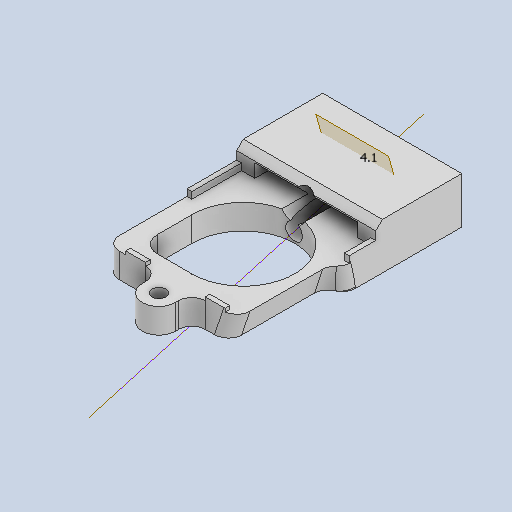
# Autodesk Inventor part: chamber bottom seal plate
Saved by Autodesk Inventor 2023.3 (Build 273359000, 359)
## iProperties
Created: 2023-03-28
Part Number: chamber bottom seal plate
Material: Generic
Document SubType Name: Modeling
Designer: splath
Density: 1 g/cm^3
Appearance: Default
Author: splath
Autodesk Inventor part; units mm, degrees
ref_plane "YZ Plane" through (0, 0, 0) normal (1, 0, 0) x (0, 1, 0)
ref_plane "XZ Plane" through (0, 0, 0) normal (0, 1, 0) x (-1, 0, 0)
ref_plane "XY Plane" through (0, 0, 0) normal (0, 0, 1) x (1, 0, 0)
sketch "Sketch1" plane through (0, 0, 0) normal (0, 0, 1) x (1, 0, 0)
  line L0 (-29.4, 0) -> (29.4, 0) construction
  line L1 (0, -2.8) -> (0, 16.8) construction
  line L2 (-21, 14) -> (21, 14)
  line L3 (21, 14) -> (21, 0)
  line L4 (21, 0) -> (-21, 0)
  line L5 (-21, 0) -> (-21, 14)
  point P0 (0, 0)
  dimension "d0" = 42
  dimension "d1" = 14
  constraints: 8 end point, 2 parallel, 1 horizontal, 1 midpoint, 1 perpendicular
  measures "d0" distance of L2.start L2.end
  measures "d1" distance of L2.end L3.end
extrude "Extrusion1" add sketch "Sketch1" along normal blind 65.5
sketch "Sketch2" plane through (0, 0, 0) normal (0, 0, -1) x (-1, 0, 0)
  line L0 (-11.5, 5) -> (11.5, 5) construction
  line L1 (0, -2.8) -> (0, 16.8) construction
  line L2 (-21, 14) -> (21, 14) construction
  line L3 (0, 5) -> (0, 0) construction
  dimension "d5" = 9
  dimension "d6" = 23
  constraints: 4 end point, 2 coincident, 1 horizontal, 1 midpoint, 1 vertical
  measures "d5" distance between parallel lines of L2 L0
  measures "d6" distance of L0.start L0.end
hole "Hole1" at (-11.5, 5, 0) at (11.5, 5, 0) direction (0, 0, 1) diameter 2.95 depth 8 tip angle 118
sketch "Sketch4" plane through (-21, 14, 0) normal (0, 1, 0) x (1, 0, 0)
  line L0 (42, 0) -> (0, 0) construction
  line L1 (0, 0) -> (0, -65.5) construction
  line L2 (42, -65.5) -> (0, -65.5) construction
  line L3 (42, 0) -> (42, -65.5) construction
  line L4 (0, -26) -> (42, -26)
  line L5 (42, -26) -> (42, -65.5)
  line L6 (42, -65.5) -> (0, -65.5)
  line L7 (0, -65.5) -> (0, -26)
  point P0 (21, 0)
  dimension "d22" = 26
  constraints: 8 end point, 3 collinear, 2 parallel, 1 horizontal, 1 perpendicular
  measures "d22" distance between parallel lines of L0 L4
extrude "Extrusion2" cut sketch "Sketch4" against normal blind 4.5
sketch "Sketch5" plane through (-21, 0, 0) normal (0, -1, 0) x (1, 0, 0)
  line L0 (0, 0) -> (42, 0) construction
  line L1 (42, 0) -> (42, 65.5) construction
  line L2 (0, 65.5) -> (42, 65.5) construction
  line L3 (0, 0) -> (0, 65.5) construction
  line L4 (21, 0) -> (21, 45) construction
  dimension "d25" = 45
  constraints: 2 end point, 1 vertical
  measures "d25" distance of L4.start L4.end
hole "Hole3" at (0, 0, 45) direction (0, 1, 0) diameter 31 end through all
sketch "Sketch6" plane through (-21, 9.5, 0) normal (0, 1, 0) x (1, 0, 0)
  line L0 (1.45, -64.1) -> (40.55, -64.1)
  line L1 (40.55, -64.1) -> (40.55, -26)
  line L2 (40.55, -26) -> (1.45, -26)
  line L3 (1.45, -26) -> (1.45, -64.1)
  line L4 (0, -26) -> (42, -26) construction
  line L5 (42, -26) -> (42, -65.5) construction
  line L6 (0, -65.5) -> (0, -26) construction
  line L7 (1.45, -41) -> (0, -41)
  line L8 (0, -41) -> (0, -65.5)
  line L9 (0, -65.5) -> (6, -65.5)
  line L10 (6, -65.5) -> (6, -64.1)
  line L11 (36, -64.1) -> (36, -65.5)
  line L12 (36, -65.5) -> (42, -65.5)
  line L13 (42, -65.5) -> (42, -34)
  line L14 (40.55, -34) -> (42, -34)
  line L15 (12, -65.5) -> (30, -65.5)
  line L16 (30, -65.5) -> (30, -64.1)
  line L17 (30, -64.1) -> (12, -64.1)
  line L18 (12, -64.1) -> (12, -65.5)
  line L19 (42, -65.5) -> (0, -65.5) construction
  point P0 (21, 0)
  point P1 (39, -65.5)
  point P2 (21, -64.1)
  dimension "d33" = 1.45
  dimension "d34" = 1.45
  dimension "d37" = 1.4
  dimension "d38" = 8
  dimension "d50" = 6
  dimension "d66" = 18
  dimension "d93" = 15
  constraints: 32 end point, 7 point on line, 5 parallel, 5 perpendicular, 4 collinear, 3 horizontal, 3 midpoint
  measures "d33" distance between parallel lines of L1 L5
  measures "d34" distance between parallel lines of L6 L3
  measures "d37" distance from line of point (39, -65.5) L0
  measures "d38" distance between parallel lines of L4 L14
  measures "d50" distance between parallel lines of L13 L11
  measures "d66" distance between parallel lines of L16 L18
  measures "d93" distance between parallel lines of L4 L7
extrude "Extrusion3" cut sketch "Sketch6" against normal blind 2
sketch "Sketch3" plane through (-0.5, -1, 34) normal (0, 0, 1) x (1, 0, 0)
  line L0 (-20.5, 1) -> (21.5, 1) construction
  line L1 (21.5, 1) -> (21.5, 8.5) construction
  line L2 (-20.5, 8.5) -> (-20.5, 1) construction
  line L3 (-8.5, 10.5) -> (-14.5, 10.5) projected
  line L4 (-14.5, 8.5) -> (-20.5, 8.5) projected
  line L5 (21.5, 8.5) -> (15.5, 8.5) projected
  line L6 (15.5, 8.5) -> (15.5, 10.5) projected
  line L7 (-14.5, 10.5) -> (-14.5, 8.5) projected
  line L8 (15.5, 10.5) -> (9.5, 10.5) projected
  line L9 (9.5, 10.5) -> (9.5, 8.5) projected
  line L10 (9.5, 8.5) -> (-8.5, 8.5) projected
  line L11 (-8.5, 8.5) -> (-8.5, 10.5) projected
  line L12 (0.5, 10) -> (0.5, 1) construction
  line L13 (21.5, 15) -> (-20.5, 15) construction
  dimension "d76" = 5
  constraints: 2 end point, 1 vertical
  measures "d76" distance from line of L12.start L13
hole "Hole2" at (0, 9, 34) direction (0, 0, -1) diameter 4.6 end through all counterbore diameter 7.5 counterbore depth 29
sketch "Sketch7" plane through (-21, 7.5, 0) normal (0, 1, 0) x (1, 0, 0)
  arc A0 (17.5631, -29.8859) -> (24.4369, -29.8859) centre (21, -45) ccw construction
  line L0 (2.9, -45) -> (39.1, -45) construction
  line L1 (0, -65.5) -> (0, -41) construction
  point P0 (21, 0)
  point P1 (21, -45)
  dimension "d49" = 2.9
  constraints: 2 coincident, 2 end point, 1 horizontal, 1 midpoint
  measures "d49" distance from line of L1 L0.start
feature "Snap Fit1" [suppressed]
fillet "Fillet1" [suppressed]
sketch "Sketch8" plane through (-21, 9.5, 0) normal (0, 1, 0) x (1, 0, 0)
  line L0 (-3.5583, -70.8259) -> (42.547, -70.8259)
  line L1 (42.547, -70.8259) -> (42.547, -58.9679)
  line L2 (42.547, -58.9679) -> (-3.5583, -58.9679)
  line L3 (-3.5583, -58.9679) -> (-3.5583, -70.8259)
  point P0 (21, 0)
  constraints: 8 end point, 2 parallel, 1 horizontal, 1 perpendicular
extrude "Extrusion4" cut sketch "Sketch8" against normal blind 1
sketch "Sketch9" plane through (-21, 0, 0) normal (0, -1, 0) x (1, 0, 0)
  line L0 (0, 65.5) -> (42, 65.5) construction
  line L1 (16, 65.5) -> (16, 70.5)
  arc A0 (26, 70.5) -> (16, 70.5) centre (21, 70.5) ccw
  line L2 (26, 70.5) -> (26, 65.5)
  line L3 (16, 65.5) -> (26, 65.5)
  point P0 (21, 0)
  point P1 (21, 65.5)
  dimension "d54" = 5
  dimension "d55" = 10
  constraints: 6 end point, 2 midpoint, 2 point on circle, 2 point on line, 2 tangent, 1 centre point, 1 collinear, 1 perpendicular, 1 vertical
  measures "d54" distance of L2.start L2.end
  measures "d55" distance between parallel lines of L1 L2
extrude "Extrusion5" add sketch "Sketch9" against normal up to surface (7.5 mm away)
sketch "Sketch10" plane through (-21, 0, 0) normal (0, -1, 0) x (1, 0, 0)
  arc A0 (26, 70.5) -> (16, 70.5) centre (21, 70.5) ccw construction
  point P0 (21, 0)
  constraints: 1 coincident
hole "Hole4" at (0, 0, 70.5) direction (0, 1, 0) diameter 4.2 end through all counterbore diameter 5.7 counterbore depth 4.2
fillet "Fillet2" radius 4 2 edges at (5, 3.75, 65.5) (-5, 3.75, 65.5)
sketch "Sketch11" plane through (0, 0, 0) normal (1, 0, 0) x (0, 1, 0)
  line L0 (7.5, 34) -> (7.5, 65.5) construction
  line L1 (11.6, 26) -> (7.5, 26)
  line L2 (7.5, 26) -> (7.5, 21.9)
  line L3 (7.5, 21.9) -> (11.6, 26)
  line L4 (9.5, 26) -> (14, 26) construction
  point P0 (0, 0)
  dimension "d68" = 4.1
  dimension "d69" = 45
  constraints: 6 end point, 2 collinear, 1 horizontal, 1 perpendicular
  measures "d68" distance from line of L2 L1.start
  measures "d69" angle of L4 L3
extrude "Extrusion6" cut sketch "Sketch11" along normal mid plane 31
chamfer "Chamfer1" distance 2 angle 45 1 edges at (0, 14, 26)
chamfer "Chamfer2" [suppressed]
sketch "Sketch12" plane through (-21, 0, 0) normal (0, -1, 0) x (1, 0, 0)
  arc A0 (36.5, 45) -> (36.5, 45) centre (21, 45) ccw construction
  line L0 (5.5, 45) -> (5.5, 55.5)
  line L1 (10.5, 60.5) -> (21, 60.5)
  line L2 (21, 60.5) -> (5.5, 45)
  arc A1 (10.5, 60.5) -> (5.5, 55.5) centre (10.5, 55.5) ccw
  point P0 (21, 0)
  point P1 (5.5, 60.5)
  dimension "d83" = 15.5
  dimension "d84" = 5
  dimension "d92" = 45
  constraints: 6 end point, 4 point on circle, 3 tangent, 2 point on line, 1 centre point, 1 horizontal, 1 vertical
  measures "d83" distance of L0.start point (5.5, 60.5)
  measures "d84" radius of A1
  measures "d92" angle of L2 L1
extrude "Extrusion7" cut sketch "Sketch12" against normal through all
sketch "Sketch13" plane through (0, 0, 65.5) normal (0, 0, 1) x (1, 0, 0)
  line L0 (9, 0) -> (21, 0) construction
  line L1 (21, 0) -> (21, 7.5) construction
  line L2 (16, 0) -> (18.5, 7.5)
  line L3 (21, 7.5) -> (21, 0)
  line L4 (21, 0) -> (16, 0)
  line L5 (21, 7.5) -> (15, 7.5) construction
  line L6 (18.5, 7.5) -> (21, 7.5)
  point P0 (0, 0)
  dimension "d87" = 5
  dimension "d91" = 2.5
  constraints: 8 end point, 3 collinear, 1 point on line
  measures "d87" distance from line of L1 L2.start
  measures "d91" distance from line of L1 L2.end
extrude "Extrusion8" cut sketch "Sketch13" against normal blind 30
fillet "Fillet3" radius 4 4 edges at (17.25, 3.75, 35.5) (17.25, 3.75, 65.5) (21, 3.75, 35.5) (-21, 3.75, 65.5)
sketch "Sketch15" plane through (0, 0, 0) normal (1, 0, 0) x (0, 1, 0)
  line L0 (12.75, 5) -> (5.25, 5) projected
  line L1 (12.75, 5) -> (12.75, 9.1) construction
  line L2 (12.75, 9.1) -> (5.25, 9.1) construction
  line L3 (9, 9.1) -> (-12.0434, 82.9693) construction
  point P0 (0, 0)
  dimension "d99" = 4.1
  constraints: 6 end point, 1 coincident, 1 horizontal, 1 midpoint
  measures "d99" distance of L0.start L1.end
ref_plane "Work Plane2" through (0, 9, 9.1) normal (0, -0.2739731, 0.9617374) x (1, 0, 0)
hole "Hole5" at (0, 9, 9.1) direction (0, -0.2739731, 0.9617374) diameter 5 end through all
sketch "Sketch14" plane through (0, -15.8521, 45) normal (0, 0, -1) x (0, 1, 0)
  line L0 (23.3521, 15.5) -> (18.3521, 15.5) projected
  line L1 (15.8521, 17.7054) -> (15.8521, 21) projected
  line L2 (15.8521, 17.7054) -> (15.8521, 14.1186) projected
  line L3 (15.8521, 14.1186) -> (15.8521, -15.5) projected
  line L4 (15.8521, -15.5) -> (15.8521, -10.5) projected
  line L5 (15.8521, -10.5) -> (15.8521, 0) projected
  line L6 (15.8521, 0) -> (15.8521, 14) projected
  line L7 (15.8521, 9.3352) -> (15.8521, 14) projected
  line L8 (15.8521, 9) -> (15.8521, 9.3352) projected
  line L9 (15.8521, 5) -> (15.8521, 9) projected
  line L10 (15.8521, 5) -> (15.8521, -5) projected
  line L11 (15.8521, -9) -> (15.8521, -5) projected
  line L12 (15.8521, -17) -> (15.8521, -9) projected
  line L13 (15.8521, -21) -> (15.8521, -17) projected
  line L14 (15.8521, -21) -> (15.8521, 21) projected
  line L15 (15.8521, -2.85) -> (15.8521, 2.85) projected
  line L16 (20.2958, 15.5) -> (15.8521, 12.8338)
  line L17 (15.8521, 14) -> (23.3521, 18.5) projected
  line L18 (16.6711, 14.4914) -> (15.8521, 14) projected
  line L19 (23.3521, 18.5) -> (16.6711, 14.4914) projected
  point P0 (15.8521, 0)
  dimension "d96" = 1
  constraints: 2 end point, 2 point on line, 1 parallel
  measures "d96" distance between parallel lines of L16 L17
body "Solid1"
